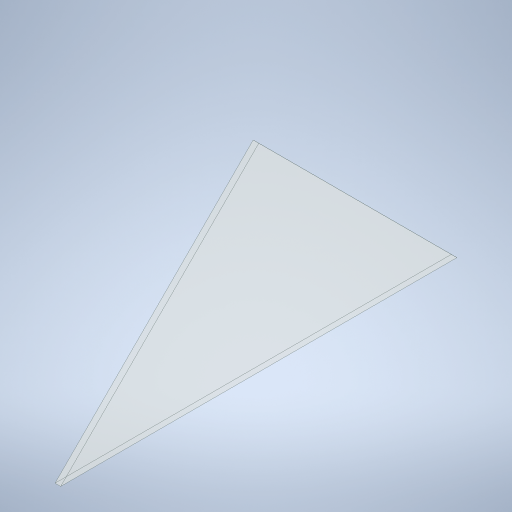
# Autodesk Inventor part: Gable
Saved by Autodesk Inventor 2024 (Build 280153000, 153)
## iProperties
Created: 2023-05-19
Part Number: Gable
Material: Wood (Southern Pine)
Document SubType Name: Modeling
Designer: Tom
Density: 0.420735 g/cm^3
Appearance: Clear
Author: Tom
Autodesk Inventor part; units mm, degrees
ref_plane "YZ Plane" through (0, 0, 0) normal (1, 0, 0) x (0, 1, 0)
ref_plane "XZ Plane" through (0, 0, 0) normal (0, 1, 0) x (-1, 0, 0)
ref_plane "XY Plane" through (0, 0, 0) normal (0, 0, 1) x (1, 0, 0)
sketch "Sketch1" plane through (0, 0, 0) normal (1, 0, 0) x (0, 1, 0)
  line L0 (0, 3810) -> (3810, 0)
  line L1 (3810, 0) -> (0, -3810)
  line L2 (0, -3810) -> (0, 3810)
  point P0 (0, 0)
  point P1 (0, 0)
  dimension "d1" = 7620
  dimension "d2" = 45
  constraints: 6 end point, 1 coincident, 1 midpoint, 1 perpendicular, 1 vertical
  measures "d1" distance of L1.end L0.start
  measures "d2" angle of L2 L0
extrude "Extrusion1" add sketch "Sketch1" along normal blind 107.95
body "Solid1"
